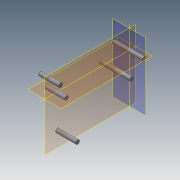
# Autodesk Inventor part: HbFingerPosture_flex02
Saved by Autodesk Inventor 2015 SP1 (Build 190203100, 203)
## iProperties
Created: 2015-02-13
Part Number: HbFingerPosture_flex02
Material: 一般
Document SubType Name: Modeling
Designer: Yamaura
Density: 1 g/cm^3
Appearance: 既定
Author: Yamaura
Autodesk Inventor part; units mm, degrees
sketch "スケッチ1" plane through (0, 0, 0) normal (1, 0, 0) x (0, 1, 0)
  circle A0 centre (0, 0) radius 1
  circle A1 centre (-36.4, 0) radius 1
  circle A2 centre (-30.8515, -21.8051) radius 1
  line L0 (-36.4, 0) -> (0, 0)
  line L1 (-30.8515, -21.8051) -> (-36.4, 0)
  line L2 (0, 0) -> (0, 70.9009)
  circle A3 centre (-6.4, -5.5) radius 1
  circle A4 centre (-39.3155, 6.9971) radius 1
  line L3 (0, 0) -> (-6.4, -5.5)
  line L4 (-39.3155, 6.9971) -> (-36.4, 0)
  line L5 (-48.5786, 0) -> (9.2631, 0) projected
  line L6 (-39.3155, 6.9971) -> (-38.2495, 7.2684)
  line L7 (-36.4, 0) -> (-38.2495, 7.2684)
  line L8 (-6.4, -5.5) -> (-39.3155, 6.9971)
  line L9 (-6.4, -5.5) -> (-5.2926, 1.9178)
  line L10 (-5.2926, 1.9178) -> (-39.3155, 6.9971)
  dimension "d0" = 2
  dimension "d1" = 2
  dimension "d2" = 2
  dimension "d3" = 36.4
  dimension "d4" = 22.5
  dimension "d5" = 90
  dimension "d9" = 2
  dimension "d10" = 2
  dimension "d23" = 1.1
  dimension "d24" = 7.5
  dimension "d29" = 6.4
  dimension "d30" = 5.5
  dimension "d33" = 7.5
  dimension "d34" = 34.4
  constraints: 20 end point, 5 centre point, 2 coincident, 2 perpendicular, 2 vertical, 1 collinear
  measures "d0" diameter of A0
  measures "d1" diameter of A1
  measures "d2" diameter of A2
  measures "d3" distance of L0.start L0.end
  measures "d4" distance of L1.start L0.start
  measures "d5" angle of L0 L2
  measures "d9" diameter of A3
  measures "d10" diameter of A4
  measures "d23" distance from line of L1 A4.centre
  measures "d24" distance of L0.start L6.end
  measures "d29" horizontal distance of L0.end L3.end
  measures "d30" vertical distance of L0.end L3.end
  measures "d33" distance of L3.end L9.end
  measures "d34" distance of L9.end L4.start
extrude "押し出し1" add sketch "スケッチ1" along normal mid plane 10 contours L5 L2 A0 | A0 L3 L5 | L2 L0 A0 | A0 L0 L3 | L3 L9 A3 | A3 L8 L3 | L9 L8 A3 | L0 L7 A1 | A1 L1 L0 | L7 L4 A1 | A1 L5 L1 | L5 A1 L4 | L8 L10 A4 | A4 L4 L8 | L10 L6 A4 | A4 L6 L4 | A2
offset faces "サイズ1" outward 2.5 faces at (5, 0.5848, -0.397) (-5, 0.5848, -0.397) (5, -6.7236, -5.5798) (-5, -6.0764, -5.4202)
